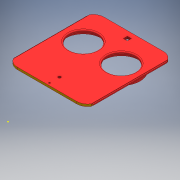
# Autodesk Inventor part: tapacuerpo
Saved by Autodesk Inventor 2019 (Build 230136000, 136)
## iProperties
Created: 2018-05-24
Part Number: tapacuerpo
Material: Genérico
Document SubType Name: Sheet Metal
Designer: USER
Density: 1 g/cm^3
Sheet Metal Rule: Por defecto_mm
Appearance: Oro
Author: USER
Autodesk Inventor part; units mm, degrees
sketch "Sketch1" plane through (0, 0, 0) normal (0, 0, 1) x (1, 0, 0)
  line L0 (20, 0) -> (130, 0)
  line L1 (150, 20) -> (150, 140)
  line L2 (130, 160) -> (20, 160)
  line L3 (0, 140) -> (0, 20)
  arc A0 (20, 160) -> (0, 140) centre (20, 140) ccw
  arc A1 (150, 140) -> (130, 160) centre (130, 140) ccw
  arc A2 (130, 0) -> (150, 20) centre (130, 20) ccw
  arc A3 (0, 20) -> (20, 0) centre (20, 20) ccw
  point P0 (0, 0)
  point P1 (150, 160)
  point P2 (150, 0)
  point P3 (0, 160)
  dimension "d443" = 160
  dimension "d444" = 150
  constraints: 8 end point, 8 point on circle, 8 point on line, 8 tangent, 4 centre point, 3 equal radius, 2 parallel, 1 horizontal, 1 perpendicular
  measures "d443" distance between parallel lines of L0 L2
  measures "d444" distance between parallel lines of L3 L1
extrude "Extrusion1" add sketch "Sketch1" along normal blind 95
sketch "Sketch5" plane through (0, 0, 95) normal (0, 0, 1) x (1, 0, 0)
  line L0 (130, 157) -> (20, 157)
  arc A0 (20, 157) -> (3, 140) centre (20, 140) ccw
  line L1 (3, 140) -> (3, 20)
  arc A1 (3, 20) -> (20, 3) centre (20, 20) ccw
  line L2 (20, 3) -> (130, 3)
  arc A2 (130, 3) -> (147, 20) centre (130, 20) ccw
  line L3 (147, 20) -> (147, 140)
  arc A3 (147, 140) -> (130, 157) centre (130, 140) ccw
  point P0 (0, 0)
  point P1 (0, 165)
  point P2 (150, 165)
  point P3 (0, 160)
  point P4 (150, 160)
  point P5 (150, 0)
  dimension "d456" = 160
  dimension "d457" = 150
  dimension "d458" = 160
  dimension "d459" = 150
  constraints: 8 end point, 8 point on circle, 4 centre point, 2 perpendicular
  measures "d456" distance of point (0, 0) point (0, 160)
  measures "d457" distance of point (0, 160) point (150, 160)
  measures "d458" distance of point (150, 160) point (150, 0)
  measures "d459" distance of point (150, 0) point (0, 0)
extrude "Extrusion2" cut sketch "Sketch5" against normal blind 92
sketch "Sketch7" plane through (0, 20, 0) normal (-1, 0, 0) x (0, 0, 1)
  circle A0 centre (47.5, 110) radius 7.8
  point P0 (95, 120)
  dimension "d455" = 15.6
  constraints: 1 centre point
  measures "d455" diameter of A0
extrude "Extrusion4" cut sketch "Sketch7" against normal blind 98
sketch "Boceto12" plane through (20, 0, 0) normal (0, -1, 0) x (1, 0, 0)
  circle A0 centre (81.375, 48) radius 12
  circle A1 centre (28.625, 48) radius 12
  constraints: 2 centre point
extrude "Extrusión6" cut sketch "Boceto12" against normal blind 5
sketch "Boceto36" plane through (20, 160, 0) normal (0, 1, 0) x (1, 0, 0)
  circle A0 centre (55, -47.7801) radius 15
  dimension "d388" = 30
  constraints: 1 centre point
  measures "d388" diameter of A0
extrude "Extrusión17" cut sketch "Boceto36" against normal blind 6
ref_plane "Plano de trabajo1" through (0, 0, -50) normal (0, 0, -1) x (-1, 0, 0)
ref_plane "Plano de trabajo4" through (203.75, 20, 0) normal (-1, 0, 0) x (0, 0, 1)
ref_plane "Plano de trabajo5" through (200, 20, 0) normal (1, 0, 0) x (0, 0, -1)
ref_plane "Plano de trabajo6" through (20, 210, 0) normal (0, 1, 0) x (1, 0, 0)
sketch "Boceto57" plane through (150, 20, 0) normal (1, 0, 0) x (0, 0, -1)
  circle A0 centre (-47.5, 110) radius 7.8
  dimension "d453" = 15.6
  constraints: 1 centre point
  measures "d453" diameter of A0
extrude "Extrusión26" cut sketch "Boceto57" against normal blind 10
sketch "Boceto61" plane through (0, 0, 0) normal (0, 0, -1) x (-1, 0, 0)
  circle A0 centre (-75, 128.3417) radius 7.5
  circle A1 centre (-74.9977, 103.4764) radius 7.5
  circle A2 centre (-74.9673, 78.5161) radius 7.5
  dimension "d399" = 15
  constraints: 3 centre point
  measures "d399" diameter of A0
extrude "Extrusión28" add sketch "Boceto61" along normal blind 4
sketch "Boceto64" plane through (20, 160, 0) normal (0, 1, 0) x (1, 0, 0)
  circle A0 centre (12, -12) radius 1.5
  circle A1 centre (98, -12) radius 1.5
  circle A2 centre (12, -83) radius 1.5
  circle A3 centre (98, -83) radius 1.5
  dimension "d417" = 3
  dimension "d418" = 3
  dimension "d468" = 3
  dimension "d469" = 3
  constraints: 4 centre point
  measures "d417" diameter of A0
  measures "d418" diameter of A1
  measures "d468" diameter of A2
  measures "d469" diameter of A3
extrude "Extrusión30" cut sketch "Boceto64" against normal blind 20
sketch "Boceto65" plane through (20, 0, 0) normal (0, -1, 0) x (1, 0, 0)
  circle A0 centre (14.995, 99.7655) radius 2.5
  circle A1 centre (94.995, 99.7655) radius 2.5
  circle A2 centre (14.995, 19.7655) radius 2.5
  circle A3 centre (94.995, 19.7655) radius 2.5
  constraints: 4 centre point
extrude "Extrusión31" cut sketch "Boceto65" against normal blind 10
sketch "Boceto66" plane through (20, 0, 0) normal (0, -1, 0) x (1, 0, 0)
  circle A0 centre (28.625, 48) radius 12 projected
  circle A1 centre (28.625, 48) radius 21
  circle A2 centre (81.375, 48) radius 12 projected
  circle A3 centre (81.375, 48) radius 21
  point P0 (-20, 0)
  dimension "d474" = 42
  dimension "d475" = 42
  constraints: 2 centre point, 2 coincident
  measures "d474" diameter of A1
  measures "d475" diameter of A3
extrude "Extrusión32" cut sketch "Boceto66" against normal blind 10
sketch "Boceto67" plane through (20, 3, 95) normal (0, 1, 0) x (1, 0, 0)
  circle A0 centre (28.625, 47) radius 21 projected
  circle A1 centre (28.625, 47) radius 21
  circle A2 centre (28.625, 47) radius 25
  point P0 (-20, 95)
  dimension "d478" = 42
  dimension "d479" = 50
  constraints: 2 centre point, 2 coincident
  measures "d478" diameter of A1
  measures "d479" diameter of A2
extrude "Extrusión33" add sketch "Boceto67" along normal blind 6
sketch "Boceto68" plane through (20, 3, 95) normal (0, 1, 0) x (1, 0, 0)
  circle A0 centre (81.375, 47) radius 21 projected
  circle A1 centre (81.375, 47) radius 25
  point P0 (-20, 95)
  dimension "d482" = 50
  constraints: 1 centre point, 1 coincident
  measures "d482" diameter of A1
extrude "Extrusión34" add sketch "Boceto68" along normal blind 6
fillet "Empalme1" radius 2 3 edges at (82.5, 128.3417, -4) (82.4977, 103.4764, -4) (82.4673, 78.5161, -4)
sketch "Boceto69" plane through (20, 160, 0) normal (0, 1, 0) x (1, 0, 0)
  line L0 (12, -22.2801) -> (82, -22.2801) projected
  line L1 (82, -22.2801) -> (82, -62.2801) projected
  line L2 (12, -62.2801) -> (12, -22.2801) projected
  line L3 (82, -62.2801) -> (12, -62.2801) projected
  point P0 (-20, 0)
extrude "Extrusión35" cut sketch "Boceto69" against normal blind 10
sketch "Boceto70" plane through (20, 3, 95) normal (0, 1, 0) x (1, 0, 0)
  point P0 (-20, 95)
sketch "Boceto71" plane through (20, 3, 95) normal (0, 1, 0) x (1, 0, 0)
  circle A0 centre (81.375, 47) radius 25 projected
  circle A1 centre (28.625, 47) radius 25 projected
  circle A2 centre (14.995, 75.2345) radius 2.5 projected
  circle A3 centre (94.995, 75.2345) radius 2.5 projected
  line L0 (110, 0) -> (0, 0) projected
  line L1 (110, 0) -> (110, 92) projected
  line L2 (110, 92) -> (0, 92) projected
  line L3 (0, 0) -> (0, 92) projected
  point P0 (-20, 95)
extrude "Extrusión36" add sketch "Boceto71" along normal up to surface (6 mm away)
sketch "Boceto72" plane through (147, 20, 95) normal (-1, 0, 0) x (0, 0, 1)
  circle A0 centre (-47.5, 110) radius 7.8 projected
  line L0 (-47.5, 110) -> (-47.5, 126.557)
  line L1 (-47.5, 126.557) -> (-53.5, 126.557)
  line L2 (-53.5, 126.557) -> (-41.5, 126.557)
  line L3 (-53.5, 126.557) -> (-41.5, 126.557)
  line L4 (-41.5, 126.557) -> (-41.5, 131.557)
  line L5 (-41.5, 131.557) -> (-53.5, 131.557)
  line L6 (-53.5, 131.557) -> (-53.5, 126.557)
  line L7 (-47.5, 126.557) -> (-47.5, 115.307)
  line L8 (-47.5, 115.307) -> (-36.0059, 115.307)
  line L9 (-47.5, 120.614) -> (-47.5, 104.057)
  line L10 (-47.5, 104.057) -> (-53.5, 104.057)
  line L11 (-53.5, 104.057) -> (-41.5, 104.057)
  line L12 (-53.5, 104.057) -> (-41.5, 104.057)
  line L13 (-41.5, 104.057) -> (-41.5, 99.057)
  line L14 (-41.5, 99.057) -> (-53.5, 99.057)
  line L15 (-53.5, 99.057) -> (-53.5, 104.057)
  line L16 (-47.5, 104.057) -> (-47.5, 115.307)
  point P0 (-95, -20)
  dimension "d490" = 16.557
  dimension "d491" = 6
  dimension "d492" = 12
  dimension "d493" = 12
  dimension "d494" = 5
  dimension "d497" = 11.25
  constraints: 34 end point, 7 symmetric about line, 4 point on line, 2 horizontal, 2 parallel, 2 perpendicular, 1 vertical
  measures "d490" distance of L0.start L0.end
  measures "d491" distance of L0.end L1.end
  measures "d492" distance of L1.end L2.end
  measures "d493" distance of L5.end L4.end
  measures "d494" distance of L4.end L3.end
  measures "d497" distance of L0.end L7.end
extrude "Extrusión37" add sketch "Boceto72" along normal blind 9 contours L1 L6 L5 L4 L2
extrude "Extrusión38" add sketch "Boceto72" along normal up to surface (9 mm away) contours L11 L13 L14 L15 L10 A0 | A0 L10 L11
sketch "Boceto73" plane through (0, 0, 95) normal (0, 0, 1) x (1, 0, 0)
  arc A0 (150, 140) -> (130, 160) centre (130, 140) ccw projected
  line L0 (130, 160) -> (150, 160)
  line L1 (150, 160) -> (150, 140)
  point P0 (0, 0)
  constraints: 4 end point, 1 horizontal, 1 perpendicular
extrude "Extrusión39" cut sketch "Boceto73" against normal blind 1200
ref_plane "Plano de trabajo20" through (75, 0, 0) normal (1, 0, 0) x (0, 1, 0)
mirror "Simetría1" about plane through (75, 0, 0) normal (1, 0, 0) of "Extrusión37", "Extrusión38"
mirror "Simetría2" about plane through (75, 0, 0) normal (1, 0, 0) of "Extrusión39"
sketch "Boceto74" plane through (138, 20, 95) normal (-1, 0, 0) x (0, 0, 1)
  arc A0 (-48, 129.616) -> (-47, 129.616) centre (-47.5, 128.75) ccw projected
  circle A1 centre (-47.5, 128.75) radius 1
  point P0 (-95, -20)
  constraints: 1 coincident, 3 other
extrude "Extrusión40" cut sketch "Boceto74" along normal blind 133 and the other way blind 8
sketch "Boceto75" plane through (138, 119.057, 41.5) normal (-1, 0, 0) x (0, 0, 1)
  arc A0 (6.5, 1.827) -> (5.5, 1.827) centre (6, 2.693) ccw projected
  circle A1 centre (6, 2.693) radius 1
  point P0 (-41.5, -119.057)
  dimension "d507" = 2
  constraints: 1 centre point, 1 coincident
  measures "d507" diameter of A1
extrude "Extrusión41" cut sketch "Boceto75" along normal blind 134 and the other way blind 9
sketch "Boceto76" plane through (0, 0, 95) normal (0, 0, 1) x (1, 0, 0)
  line L0 (150, 20) -> (150, 140) projected
  line L1 (147, 140) -> (147, 20) projected
  line L2 (3, 20) -> (3, 140) projected
  line L3 (0, 140) -> (0, 20) projected
  line L4 (0, 140) -> (3, 140)
  line L5 (0, 20) -> (3, 20)
  line L6 (147, 20) -> (150, 20)
  line L7 (147, 140) -> (147, 20) projected
  line L8 (147, 140) -> (150, 140)
  point P0 (0, 0)
  constraints: 8 end point, 2 equal length, 1 horizontal, 1 perpendicular
extrude "Extrusión42" add sketch "Boceto76" along normal blind 4
sketch "Boceto77" plane through (147, 20, 3) normal (-1, 0, 0) x (0, 0, 1)
  line L0 (96, 0) -> (96, 120) projected
  line L1 (96, 120) -> (95, 120)
  line L2 (92, 120) -> (96, 120) projected
  line L3 (95, 120) -> (93, 120)
  line L4 (93, 120) -> (93, 0)
  line L5 (93, 0) -> (95, 0)
  line L6 (95, 0) -> (95, 120)
  point P0 (-3, -20)
  dimension "d514" = 1
  dimension "d515" = 2
  constraints: 10 end point, 2 parallel, 1 horizontal, 1 perpendicular, 1 point on line
  measures "d514" distance of L0.end L1.end
  measures "d515" distance of L5.end L4.end
extrude "Extrusión43" cut sketch "Boceto77" against normal blind 1.5
extrude "Extrusión44" cut sketch "Boceto77" along normal blind 1.5 from surface at 144
sketch "Boceto78" plane through (0, 0, 95) normal (0, 0, 1) x (1, 0, 0)
  line L0 (20, 9) -> (130, 9) projected
  line L1 (75, 9) -> (75, 0)
  circle A0 centre (75, 4.5) radius 1.5
  point P0 (0, 0)
  dimension "d520" = 3
  constraints: 2 end point, 2 midpoint, 1 centre point, 1 vertical
  measures "d520" diameter of A0
extrude "Extrusión45" cut sketch "Boceto78" against normal blind 10
sketch "Boceto79" plane through (0, 0, 95) normal (0, 0, 1) x (1, 0, 0)
  line L0 (130, 160) -> (20, 160) projected
  arc A0 (20, 160) -> (0, 140) centre (20, 140) ccw projected
  line L1 (0, 140) -> (0, 20) projected
  arc A1 (0, 20) -> (20, 0) centre (20, 20) ccw projected
  line L2 (20, 0) -> (130, 0) projected
  arc A2 (130, 0) -> (150, 20) centre (130, 20) ccw projected
  line L3 (150, 20) -> (150, 140) projected
  arc A3 (150, 140) -> (130, 160) centre (130, 140) ccw projected
  point P0 (0, 0)
extrude "Extrusión46" add sketch "Boceto79" along normal blind 4
sketch "Boceto80" plane through (75, 0, 0) normal (1, 0, 0) x (0, 1, 0)
  line L0 (140, 99) -> (20, 99) projected
  line L1 (20, 95) -> (20, 3) projected
  line L2 (20, 99) -> (20, 95)
  line L3 (-19.9561, 95) -> (216.2183, 95)
  line L4 (216.2183, 95) -> (216.2183, -18.3068)
  line L5 (216.2183, -18.3068) -> (-19.9561, -18.3068)
  line L6 (-19.9561, -18.3068) -> (-19.9561, 95)
  point P0 (0, 0)
  dimension "d525" = 4
  constraints: 10 end point, 2 parallel, 1 collinear, 1 horizontal, 1 perpendicular
  measures "d525" distance of L0.end L1.start
extrude "Extrusión47" cut sketch "Boceto80" along normal mid plane 300
sketch "Boceto81" plane through (150, 20, 99) normal (1, 0, 0) x (0, 0, -1)
  line L0 (4, 140) -> (4, 120) projected
  line L1 (4, 140) -> (4, 137)
  line L2 (4, 137) -> (3, 137)
  line L3 (3, 137) -> (3, 138.5)
  line L4 (3, 138.5) -> (1, 138.5)
  line L5 (1, 138.5) -> (1, 137)
  line L6 (1, 137) -> (0, 137)
  line L7 (0, 140) -> (0, 120) projected
  line L8 (0, 137) -> (0, 140)
  line L9 (0, 140) -> (4, 140)
  line L10 (4, 0) -> (4, 120) projected
  line L11 (4, 60) -> (-16.1997, 60)
  line L12 (4, -20) -> (4, 0)
  line L13 (4, -20) -> (4, -17)
  line L14 (4, -17) -> (3, -17)
  line L15 (3, -17) -> (3, -18.5)
  line L16 (3, -18.5) -> (1, -18.5)
  line L17 (1, -18.5) -> (1, -17)
  line L18 (1, -17) -> (0, -17)
  line L19 (0, -20) -> (0, 0)
  line L20 (0, -17) -> (0, -20)
  line L21 (0, -20) -> (4, -20)
  point P0 (99, -20)
  dimension "d528" = 3
  dimension "d529" = 1
  dimension "d530" = 1.5
  dimension "d531" = 2
  dimension "d532" = 1.5
  dimension "d533" = 1
  constraints: 38 end point, 9 symmetric about line, 6 point on line, 4 perpendicular, 1 collinear, 1 horizontal, 1 midpoint
  measures "d528" distance of L0.start L1.end
  measures "d529" distance of L1.end L2.end
  measures "d530" distance of L2.end L3.end
  measures "d531" distance of L3.end L4.end
  measures "d532" distance of L4.end L5.end
  measures "d533" distance of L5.end L6.end
sketch "Boceto83" plane through (20, 0, 99) normal (0, -1, 0) x (1, 0, 0)
  line L0 (130, -4) -> (110, -4) projected
  line L1 (130, -4) -> (127, -4)
  line L2 (127, -4) -> (127, -3)
  line L3 (127, -3) -> (128.5, -3)
  line L4 (128.5, -3) -> (128.5, -1)
  line L5 (128.5, -1) -> (127, -1)
  line L6 (127, -1) -> (127, 0)
  line L7 (130, 0) -> (110, 0) projected
  line L8 (127, 0) -> (130, 0)
  line L9 (130, -4) -> (130, 0) projected
  line L10 (130, 0) -> (130, -4)
  line L11 (0, 0) -> (110, 0) projected
  line L12 (55, 0) -> (55, -2)
  line L13 (-20, -4) -> (0, -4)
  line L14 (-20, -4) -> (-17, -4)
  line L15 (-17, -4) -> (-17, -3)
  line L16 (-17, -3) -> (-18.5, -3)
  line L17 (-18.5, -3) -> (-18.5, -1)
  line L18 (-18.5, -1) -> (-17, -1)
  line L19 (-17, -1) -> (-17, 0)
  line L20 (-20, 0) -> (0, 0)
  line L21 (-17, 0) -> (-20, 0)
  line L22 (-20, -4) -> (-20, 0)
  line L23 (-20, 0) -> (-20, -4)
  point P0 (-20, -99)
  dimension "d540" = 3
  dimension "d541" = 1
  dimension "d542" = 1.5
  dimension "d543" = 2
  dimension "d544" = 1.5
  constraints: 40 end point, 9 symmetric about line, 4 perpendicular, 4 point on line, 2 vertical, 1 collinear, 1 horizontal, 1 midpoint
  measures "d540" distance of L0.start L1.end
  measures "d541" distance of L1.end L2.end
  measures "d542" distance of L2.end L3.end
  measures "d543" distance of L3.end L4.end
  measures "d544" distance of L4.end L5.end
extrude "Extrusión50" cut sketch "Boceto83" against normal blind 200
sketch "Boceto84" plane through (0, 0, 99) normal (0, 0, 1) x (1, 0, 0)
  line L0 (20, 0) -> (130, 0) projected
  line L1 (75, 0) -> (75, 4.5)
  circle A0 centre (75, 4.5) radius 1.5
  point P0 (0, 0)
  dimension "d547" = 4.5
  dimension "d548" = 3
  constraints: 2 end point, 1 centre point, 1 coincident, 1 midpoint, 1 vertical
  measures "d547" distance of L1.start L1.end
  measures "d548" diameter of A0
extrude "Extrusión51" cut sketch "Boceto84" against normal blind 200
sketch "Boceto85" plane through (0, 0, 95) normal (0, 0, -1) x (-1, 0, 0)
  circle A0 centre (-110, 102) radius 32.75
  circle A1 centre (-40, 102) radius 32.75
  circle A2 centre (-110, 102) radius 34.75
  circle A3 centre (-40, 102) radius 34.75
  point P0 (0, 0)
  dimension "d555" = 65.5
  dimension "d558" = 65.5
  dimension "d559" = 2
  dimension "d560" = 2
  constraints: 4 centre point
  measures "d555" diameter of A0
  measures "d558" diameter of A1
  measures "d559" radial gap between concentric circles of A0 A2
  measures "d560" radial gap between concentric circles of A1 A3
extrude "Extrusión52" add sketch "Boceto85" along normal blind 7
sketch "Boceto86" plane through (110, 102, 95) normal (0, 0, -1) x (-1, 0, 0)
  circle A0 centre (0, 0) radius 26.5
  circle A1 centre (70, 0) radius 26.5
  point P0 (110, -102)
  dimension "d563" = 53
  dimension "d564" = 53
  constraints: 2 centre point, 2 coincident
  measures "d563" diameter of A0
  measures "d564" diameter of A1
extrude "Extrusión53" cut sketch "Boceto86" against normal blind 8
fillet "Empalme2" radius 2 2 edges at (66.5, 102, 99) (136.5, 102, 99)
sketch "Boceto87" plane through (0, 0, 95) normal (0, 0, -1) x (-1, 0, 0)
  line L0 (-79.75, 151) -> (-75, 151)
  line L1 (-79.75, 151) -> (-79.75, 143.5)
  line L2 (-79.75, 143.5) -> (-72.25, 143.5)
  line L3 (-72.25, 143.5) -> (-72.25, 151)
  line L4 (-75, 151) -> (-72.25, 151)
  dimension "d587" = 4.75
  dimension "d593" = 7.5
  dimension "d594" = 7.5
  constraints: 10 end point, 1 horizontal, 1 perpendicular, 1 vertical
  measures "d587" distance of L0.start L0.end
  measures "d593" distance of L0.start L1.end
  measures "d594" distance of L1.end L2.end
extrude "Extrusión54" cut sketch "Boceto87" against normal blind 8
sketch "Boceto88" plane through (0, 0, 99) normal (0, 0, 1) x (1, 0, 0)
  circle A0 centre (75, 22.9196) radius 2.5
  point P0 (0, 0)
  dimension "d584" = 5
  constraints: 1 centre point
  measures "d584" diameter of A0
extrude "Extrusión55" cut sketch "Boceto88" against normal blind 10
equation "\"BendRadius\" = Thickness"
equation "\"BendReliefWidth\" = Thickness"
equation "\"BendReliefDepth\" = 0.5 * Thickness"
equation "\"CornerReliefSize\" = 4 * Thickness"
equation "\"MinimumRemnant\" = 2 * Thickness"
equation "\"TransitionRadius\" = BendRadius"
equation "\"JacobiRadiusSize\" = BendRadius"
equation "\"GapSize\" = Thickness"
equation "\"Thickness\" = 0.5"
body "Solid1"
